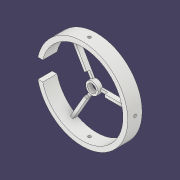
# Autodesk Inventor part: AA051
Saved by Autodesk Inventor 2017 SP1 (Build 210196100, 196)
## iProperties
Created: 2018-04-16
Part Number: AA051
Material: ABS Plastic
Document SubType Name: Modeling
Designer: Zach
Density: 1.06 g/cm^3
Appearance: CR White
Author: Zach
Autodesk Inventor part; units mm, degrees
ref_plane "YZ Plane" through (0, 0, 0) normal (1, 0, 0) x (0, 1, 0)
ref_plane "XZ Plane" through (0, 0, 0) normal (0, 1, 0) x (-1, 0, 0)
ref_plane "XY Plane" through (0, 0, 0) normal (0, 0, 1) x (1, 0, 0)
sketch "Sketch1" plane through (0, 0, 0) normal (0, 0, 1) x (1, 0, 0)
  circle A0 centre (0, 0) radius 47.5 construction
  line L0 (-46.4354, 10) -> (-46.4354, -10) construction
  circle A1 centre (0, 0) radius 42.5 construction
  line L1 (-46.4354, 10) -> (-41.3068, 10)
  line L2 (-46.4354, -10) -> (-41.3068, -10)
  arc A2 (-46.4354, -10) -> (-46.4354, 10) centre (0, 0) ccw
  arc A3 (-41.3068, -10) -> (-41.3068, 10) centre (0, 0) ccw
  circle A4 centre (0, 0) radius 4.5
  circle A5 centre (0, 0) radius 6.5
  line L3 (4.2426, 1.5) -> (47.4763, 1.5)
  line L4 (4.2426, -1.5) -> (47.4763, -1.5)
  arc A6 (4.2426, -1.5) -> (4.2426, 1.5) centre (0, 0) ccw
  arc A7 (47.4763, -1.5) -> (47.4763, 1.5) centre (0, 0) ccw
  line L5 (-3.4204, 2.9242) -> (-25.0372, 40.3657)
  line L6 (-0.8223, 4.4242) -> (-22.4391, 41.8657)
  line L7 (-0.8223, -4.4242) -> (-22.4391, -41.8657)
  line L8 (-3.4204, -2.9242) -> (-25.0372, -40.3657)
  arc A8 (-0.8223, 4.4242) -> (-3.4204, 2.9242) centre (0, 0) ccw
  arc A9 (-3.4204, -2.9242) -> (-0.8223, -4.4242) centre (0, 0) ccw
  arc A10 (-22.4391, 41.8657) -> (-25.0372, 40.3657) centre (0, 0) ccw
  arc A11 (-25.0372, -40.3657) -> (-22.4391, -41.8657) centre (0, 0) ccw
  point P0 (-46.4354, 0)
  dimension "d0" = 95
  dimension "d1" = 20
  dimension "d2" = 5
  dimension "d5" = 9
  dimension "d7" = 3
  dimension "d10" = 360
  dimension "d17" = 13
  constraints: 27 point on circle, 18 end point, 12 centre point, 5 coincident, 4 concentric, 2 vertical alignment, 1 horizontal, 1 horizontal alignment, 1 midpoint, 1 parallel, 1 perpendicular, 1 vertical, 19 other
  measures "d0" diameter of A0
  measures "d1" distance of L0.start L0.end
  measures "d2" radial gap between concentric circles of A0 A1
  measures "d5" diameter of A4
  measures "d7" distance between parallel lines of L4 L3
  measures "d17" diameter of A5
extrude "Extrusion1" add sketch "Sketch1" along normal blind 15 contours A2 L5 A3 L1 | A2 L6 A3 L5 | A2 L3 A3 L6 | L5 A4 L8 A5 | A5 L6 A4 L5 | A2 L4 A3 L3 | A5 L3 A4 L6 | L8 A4 L7 A5 | A2 L7 A3 L4 | A5 L4 A4 L3 | L7 A4 L4 A5 | L8 A2 L2 A3 | A3 L7 A2 L8
extrude "Extrusion2" add sketch "Sketch1" along normal blind 5 contours A2 L6 A3 L5 | A3 L6 A5 L5 | A5 L6 A4 L5 | A2 L4 A3 L3 | A3 L4 A5 L3 | L8 A4 L7 A5 | A5 L7 A3 L8 | A5 L4 A4 L3 | A3 L7 A2 L8
sketch "Sketch3" plane through (0, 0, 15) normal (0, 0, 1) x (1, 0, 0)
  circle A0 centre (0, 0) radius 4.5 projected
  circle A1 centre (0, 0) radius 6.5 projected
  point P0 (0, 0)
extrude "Extrusion3" cut sketch "Sketch3" against normal blind 10
sketch "Sketch4" plane through (0, 0, 5) normal (0, 0, 1) x (1, 0, 0)
  arc A0 (6.3246, 1.5) -> (-1.8632, 6.2272) centre (0, 0) ccw projected
  line L0 (42.4735, 1.5) -> (6.3246, 1.5) projected
  circle A1 centre (0, 0) radius 6.5
  circle A2 centre (0, 0) radius 13.5
  point P0 (0, 0)
  dimension "d18" = 27
  constraints: 2 coincident, 1 centre point, 3 other
  measures "d18" diameter of A2
extrude "Extrusion4" cut sketch "Sketch4" against normal blind 3
sketch "Sketch5" plane through (0, 0, 0) normal (1, 0, 0) x (0, 1, 0)
  line L0 (-10, 0) -> (10, 0) projected
  line L1 (10, 0) -> (10, 15) projected
  line L2 (-10, 15) -> (10, 15) projected
  line L3 (-10, 0) -> (-10, 15) projected
  circle A0 centre (0, 7.5) radius 1.5
  point P0 (0, 0)
  point P1 (-10, 7.5)
  point P2 (0, 0)
  dimension "d21" = 3
  constraints: 2 midpoint, 1 centre point, 1 horizontal alignment, 1 vertical alignment
  measures "d21" diameter of A0
extrude "Extrusion5" cut sketch "Sketch5" along normal through all contours A0
sketch "Sketch6" plane through (0, 0, 0) normal (0, 1, 0) x (-1, 0, 0)
  circle A0 centre (0, 7.5) radius 1.5
  point P0 (0, 0)
  dimension "d24" = 3
  dimension "d25" = 7.5
  constraints: 1 centre point, 1 vertical alignment
  measures "d24" diameter of A0
  measures "d25" distance of point (0, 0) A0.centre
extrude "Extrusion6" cut sketch "Sketch6" along normal through all both and the other way through all
body "Solid1"
